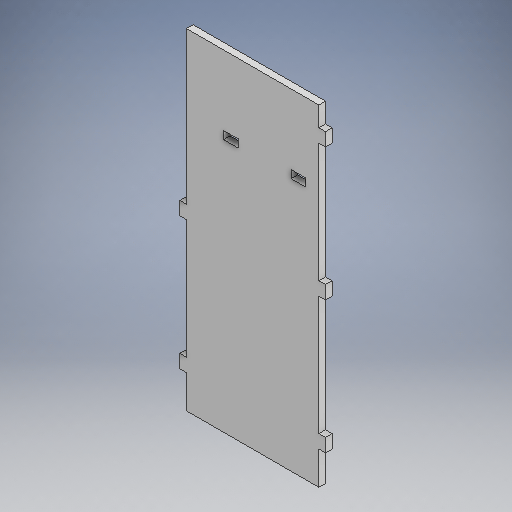
# Autodesk Inventor part: Lifting Sections back
Saved by Autodesk Inventor 2025.3 (Build 293356000, 356)
## iProperties
Created: 2026-04-06
Part Number: Lifting Sections back
Material: Generic
Document SubType Name: Modeling
Designer: user
Density: 1 g/cm^3
Appearance: Default
Author: user
Autodesk Inventor part; units mm, degrees
ref_plane "YZ Plane" through (0, 0, 0) normal (1, 0, 0) x (0, 1, 0)
ref_plane "XZ Plane" through (0, 0, 0) normal (0, 1, 0) x (-1, 0, 0)
ref_plane "XY Plane" through (0, 0, 0) normal (0, 0, 1) x (1, 0, 0)
sketch "Sketch1" plane through (0, 0, 0) normal (0, 0, 1) x (1, 0, 0)
  line L0 (-100.6151, -124.6674) -> (-100.6151, 125.3326)
  line L1 (-41.6151, -124.6674) -> (-41.6151, 125.3326) construction
  line L2 (-0.6151, -124.6674) -> (-0.6151, 73.3335)
  line L3 (-0.6151, -124.6674) -> (-100.6151, -124.6674)
  line L4 (4.3849, 110.4326) -> (-0.6151, 110.4326)
  line L5 (4.3849, 100.3326) -> (4.3849, 110.4326)
  line L6 (-0.6151, 100.3326) -> (4.3849, 100.3326)
  line L7 (4.3849, -89.5674) -> (-0.6151, -89.5674)
  line L8 (4.3849, -99.6674) -> (4.3849, -89.5674)
  line L9 (-0.6151, -99.6674) -> (4.3849, -99.6674)
  line L10 (-100.6151, 10.4326) -> (-100.6151, 0.3326)
  line L11 (-100.6151, 0.3326) -> (-0.6151, 0.3326) construction
  line L12 (-0.6151, 0.3326) -> (4.3849, 0.3326)
  line L13 (-0.6151, 0.3326) -> (4.3849, 0.3326)
  line L14 (4.3849, 0.3326) -> (4.3849, 10.4326)
  line L15 (4.3849, 0.3326) -> (4.3849, 10.4326)
  line L16 (4.3849, 10.4326) -> (-0.6151, 10.4326)
  line L17 (4.3849, 10.4326) -> (-0.6151, 10.4326)
  line L18 (-0.6151, 73.3335) -> (-0.6151, 125.3326)
  line L19 (-0.6151, 125.3326) -> (-0.6151, 75.3326)
  line L20 (-0.6151, 75.3326) -> (-100.6151, 75.3326) construction
  line L21 (-105.6151, -99.6674) -> (-105.6151, -89.5674)
  line L22 (-105.6151, -89.5674) -> (-100.6151, -89.5674)
  line L23 (-100.6151, -99.6674) -> (-105.6151, -99.6674)
  line L24 (-105.6151, 10.4326) -> (-100.6151, 10.4326)
  line L25 (-105.6151, 0.3326) -> (-105.6151, 10.4326)
  line L26 (-100.6151, 0.3326) -> (-105.6151, 0.3326)
  line L27 (-100.6151, 125.3326) -> (-0.6151, 125.3326)
  line L28 (-0.6151, 125.3326) -> (-10.6151, 125.3326)
  line L29 (-0.6151, 76.5945) -> (-0.6151, 125.3326)
  line L30 (-100.6151, 125.3326) -> (-90.6151, 125.3326)
  line L31 (-100.6151, 76.6641) -> (-100.6151, 125.3326)
  line L32 (-82.6151, 75.3326) -> (17.3849, 75.3326) construction
  line L33 (-10.6151, 72.6641) -> (-10.6151, 66.6641)
  line L34 (-21.6151, 72.6641) -> (-21.6151, 66.6641)
  line L35 (-61.6151, 72.6641) -> (-61.6151, 66.6641)
  line L36 (-72.6151, 72.6641) -> (-72.6151, 66.6641)
  line L37 (-21.6151, 72.6641) -> (-61.6151, 72.6641) construction
  line L38 (-21.6151, 66.6641) -> (-61.6151, 66.6641) construction
  line L39 (-10.6151, 66.6641) -> (-21.6151, 66.6641)
  line L40 (-10.6151, 72.6641) -> (-21.6151, 72.6641)
  line L41 (-61.6151, 72.6641) -> (-72.6151, 72.6641)
  line L42 (-61.6151, 66.6641) -> (-72.6151, 66.6641)
  line L43 (-72.6151, 66.6641) -> (-100.6151, 66.6641) construction
  line L44 (-72.6151, 72.6641) -> (-100.6151, 72.6641) construction
  point P0 (0, 0)
  point P1 (4.3849, 105.3826)
  point P2 (-10.6151, 69.6641)
  point P3 (4.3849, -94.6174)
  point P4 (4.3849, 5.3826)
  point P5 (4.3849, 5.3826)
  point P6 (-105.6151, -94.6174)
  point P7 (-105.6151, 5.3826)
  dimension "d1" = 11
  dimension "d4" = 40
  dimension "d6" = 5
  dimension "d7" = 10
  dimension "d8" = 100
  constraints: 90 end point, 12 perpendicular, 7 midpoint, 6 symmetric about line, 5 point on line, 3 vertical alignment, 2 horizontal, 1 vertical
  measures "d1" distance between parallel lines of L34 L33
  measures "d4" distance between parallel lines of L34 L35
  measures "d6" distance from line of point (4.385, 105.383) L29
  measures "d7" distance from line of L2 point (-10.615, 69.664)
  measures "d8" distance between parallel lines of L2 L0
extrude "Extrusion1" add sketch "Sketch1" along normal blind 5
body "Solid1"
